Autodesk Fusion 360 part; units mm, degrees
(part 2 of 2)
sketch "Sketch6" plane through (0, 0, 0) normal (0, 0, -1) x (1, 0, 0)
  line L0 (39, 37.5) -> (39, -37.5)
  line L1 (29, -37.5) -> (29, 37.5)
  circle A0 centre (109.2154, 0) radius 7
  circle A1 centre (-109.2154, 0) radius 7
  circle A2 centre (54.6077, 94.5833) radius 7
  circle A3 centre (54.6077, -94.5833) radius 7
  circle A4 centre (-54.6077, -94.5833) radius 7
  circle A5 centre (-54.6077, 94.5833) radius 7
  line L2 (54.6077, 109.3333) -> (-54.6077, 109.3333)
  arc A6 (-54.6077, 109.3333) -> (-67.3816, 101.9583) centre (-54.6077, 94.5833) ccw
  line L3 (-67.3816, 101.9583) -> (-121.9893, 7.375)
  arc A7 (-121.9893, 7.375) -> (-121.9893, -7.375) centre (-109.2154, 0) ccw
  line L4 (-121.9893, -7.375) -> (-67.3816, -101.9583)
  arc A8 (-67.3816, -101.9583) -> (-54.6077, -109.3333) centre (-54.6077, -94.5833) ccw
  line L5 (-54.6077, -109.3333) -> (54.6077, -109.3333)
  arc A9 (54.6077, -109.3333) -> (67.3816, -101.9583) centre (54.6077, -94.5833) ccw
  line L6 (67.3816, -101.9583) -> (121.9893, -7.375)
  arc A10 (121.9893, -7.375) -> (121.9893, 7.375) centre (109.2154, 0) ccw
  line L7 (121.9893, 7.375) -> (67.3816, 101.9583)
  arc A11 (67.3816, 101.9583) -> (54.6077, 109.3333) centre (54.6077, 94.5833) ccw
  line L8 (0, 0) -> (-123.9654, 0) construction
  circle A12 centre (-89.2154, 0) radius 2.35
  line L9 (-53.7561, -78.4378) -> (-50.1995, -84.598)
  arc A13 (-48.1643, -68.6025) -> (-50.3294, -69.8525) centre (-48.1643, -71.1025) ccw
  line L10 (-39.0159, -84.598) -> (-35.4593, -78.4378)
  arc A14 (-41.0511, -85.923) -> (-38.886, -84.673) centre (-41.0511, -83.423) ccw
  line L11 (-48.1643, -85.923) -> (-41.0511, -85.923)
  arc A15 (-53.7561, -76.0878) -> (-53.7561, -78.4378) centre (-51.7209, -77.2628) ccw
  arc A16 (-41.0511, -85.773) -> (-39.0159, -84.598) centre (-41.0511, -83.423) ccw
  line L12 (-41.0511, -68.7525) -> (-48.1643, -68.7525)
  line L13 (-53.886, -78.5128) -> (-50.3294, -84.673)
  line L14 (-35.3294, -76.0128) -> (-38.886, -69.8525)
  arc A17 (-35.3294, -78.5128) -> (-35.3294, -76.0128) centre (-37.4944, -77.2628) ccw
  arc A18 (-38.886, -69.8525) -> (-41.0511, -68.6025) centre (-41.0511, -71.1025) ccw
  circle A19 centre (-32.4026, -66.1229) radius 2.85
  line L15 (-35.4593, -76.0878) -> (-39.0159, -69.9275)
  line L16 (-48.1643, -85.773) -> (-41.0511, -85.773)
  circle A20 centre (-44.6077, -77.2628) radius 2.35
  arc A21 (-35.4593, -78.4378) -> (-35.4593, -76.0878) centre (-37.4944, -77.2628) ccw
  arc A22 (-50.3294, -84.673) -> (-48.1643, -85.923) centre (-48.1643, -83.423) ccw
  arc A23 (-53.886, -76.0128) -> (-53.886, -78.5128) centre (-51.7209, -77.2628) ccw
  line L17 (-38.886, -84.673) -> (-35.3294, -78.5128)
  line L18 (-50.1995, -69.9275) -> (-53.7561, -76.0878)
  arc A24 (-39.0159, -69.9275) -> (-41.0511, -68.7525) centre (-41.0511, -71.1025) ccw
  arc A25 (-48.1643, -68.7525) -> (-50.1995, -69.9275) centre (-48.1643, -71.1025) ccw
  line L19 (-50.3294, -69.8525) -> (-53.886, -76.0128)
  line L20 (-41.0511, -68.6025) -> (-48.1643, -68.6025)
  arc A26 (-50.1995, -84.598) -> (-48.1643, -85.773) centre (-48.1643, -83.423) ccw
  circle A27 centre (-41.0628, -61.1229) radius 2.85
  line L21 (41.0511, -85.773) -> (48.1643, -85.773)
  arc A28 (35.3294, -76.0128) -> (35.3294, -78.5128) centre (37.4944, -77.2628) ccw
  line L22 (53.7561, -76.0878) -> (50.1995, -69.9275)
  arc A29 (53.886, -78.5128) -> (53.886, -76.0128) centre (51.7209, -77.2628) ccw
  line L23 (50.3294, -84.673) -> (53.886, -78.5128)
  arc A30 (39.0159, -84.598) -> (41.0511, -85.773) centre (41.0511, -83.423) ccw
  arc A31 (53.7561, -78.4378) -> (53.7561, -76.0878) centre (51.7209, -77.2628) ccw
  line L24 (39.0159, -69.9275) -> (35.4593, -76.0878)
  line L25 (41.0511, -85.923) -> (48.1643, -85.923)
  line L26 (48.1643, -68.6025) -> (41.0511, -68.6025)
  arc A32 (50.3294, -69.8525) -> (48.1643, -68.6025) centre (48.1643, -71.1025) ccw
  arc A33 (41.0511, -68.6025) -> (38.886, -69.8525) centre (41.0511, -71.1025) ccw
  circle A34 centre (41.0628, -61.1229) radius 2.85
  line L27 (48.1643, -68.7525) -> (41.0511, -68.7525)
  line L28 (50.1995, -84.598) -> (53.7561, -78.4378)
  circle A35 centre (44.6077, -77.2628) radius 2.35
  arc A36 (50.1995, -69.9275) -> (48.1643, -68.7525) centre (48.1643, -71.1025) ccw
  arc A37 (48.1643, -85.923) -> (50.3294, -84.673) centre (48.1643, -83.423) ccw
  arc A38 (38.886, -84.673) -> (41.0511, -85.923) centre (41.0511, -83.423) ccw
  line L29 (53.886, -76.0128) -> (50.3294, -69.8525)
  line L30 (35.4593, -78.4378) -> (39.0159, -84.598)
  arc A39 (41.0511, -68.7525) -> (39.0159, -69.9275) centre (41.0511, -71.1025) ccw
  arc A40 (35.4593, -76.0878) -> (35.4593, -78.4378) centre (37.4944, -77.2628) ccw
  line L31 (35.3294, -78.5128) -> (38.886, -84.673)
  line L32 (38.886, -69.8525) -> (35.3294, -76.0128)
  arc A41 (48.1643, -85.773) -> (50.1995, -84.598) centre (48.1643, -83.423) ccw
  circle A42 centre (32.4026, -66.1229) radius 2.85
  line L33 (94.8072, -7.3353) -> (98.3638, -1.175)
  arc A43 (83.4937, -7.4103) -> (85.6588, -8.6603) centre (85.6588, -6.1603) ccw
  line L34 (92.772, 8.5103) -> (85.6588, 8.5103)
  arc A44 (94.9371, 7.4103) -> (92.772, 8.6603) centre (92.772, 6.1603) ccw
  line L35 (98.4937, 1.25) -> (94.9371, 7.4103)
  arc A45 (92.772, -8.5103) -> (94.8072, -7.3353) centre (92.772, -6.1603) ccw
  arc A46 (94.8072, 7.3353) -> (92.772, 8.5103) centre (92.772, 6.1603) ccw
  line L36 (80.067, -1.175) -> (83.6236, -7.3353)
  line L37 (94.9371, -7.4103) -> (98.4937, -1.25)
  line L38 (83.4937, 7.4103) -> (79.9371, 1.25)
  arc A47 (85.6588, 8.6603) -> (83.4937, 7.4103) centre (85.6588, 6.1603) ccw
  arc A48 (79.9371, 1.25) -> (79.9371, -1.25) centre (82.1021, 0) ccw
  circle A49 centre (73.4654, 5) radius 2.85
  line L39 (83.6236, 7.3353) -> (80.067, 1.175)
  line L40 (98.3638, 1.175) -> (94.8072, 7.3353)
  circle A50 centre (89.2154, 0) radius 2.35
  arc A51 (85.6588, 8.5103) -> (83.6236, 7.3353) centre (85.6588, 6.1603) ccw
  arc A52 (98.4937, -1.25) -> (98.4937, 1.25) centre (96.3286, 0) ccw
  arc A53 (92.772, -8.6603) -> (94.9371, -7.4103) centre (92.772, -6.1603) ccw
  line L41 (92.772, 8.6603) -> (85.6588, 8.6603)
  line L42 (85.6588, -8.5103) -> (92.772, -8.5103)
  arc A54 (80.067, 1.175) -> (80.067, -1.175) centre (82.1021, 0) ccw
  arc A55 (83.6236, -7.3353) -> (85.6588, -8.5103) centre (85.6588, -6.1603) ccw
  line L43 (85.6588, -8.6603) -> (92.772, -8.6603)
  line L44 (79.9371, -1.25) -> (83.4937, -7.4103)
  arc A56 (98.3638, -1.175) -> (98.3638, 1.175) centre (96.3286, 0) ccw
  circle A57 centre (73.4654, -5) radius 2.85
  line L45 (53.7561, 78.4378) -> (50.1995, 84.598)
  arc A58 (48.1643, 68.6025) -> (50.3294, 69.8525) centre (48.1643, 71.1025) ccw
  line L46 (39.0159, 84.598) -> (35.4593, 78.4378)
  arc A59 (41.0511, 85.923) -> (38.886, 84.673) centre (41.0511, 83.423) ccw
  line L47 (48.1643, 85.923) -> (41.0511, 85.923)
  arc A60 (53.7561, 76.0878) -> (53.7561, 78.4378) centre (51.7209, 77.2628) ccw
  arc A61 (41.0511, 85.773) -> (39.0159, 84.598) centre (41.0511, 83.423) ccw
  line L48 (41.0511, 68.7525) -> (48.1643, 68.7525)
  line L49 (53.886, 78.5128) -> (50.3294, 84.673)
  line L50 (35.3294, 76.0128) -> (38.886, 69.8525)
  arc A62 (35.3294, 78.5128) -> (35.3294, 76.0128) centre (37.4944, 77.2628) ccw
  arc A63 (38.886, 69.8525) -> (41.0511, 68.6025) centre (41.0511, 71.1025) ccw
  circle A64 centre (32.4026, 66.1229) radius 2.85
  line L51 (35.4593, 76.0878) -> (39.0159, 69.9275)
  line L52 (48.1643, 85.773) -> (41.0511, 85.773)
  circle A65 centre (44.6077, 77.2628) radius 2.35
  arc A66 (35.4593, 78.4378) -> (35.4593, 76.0878) centre (37.4944, 77.2628) ccw
  arc A67 (50.3294, 84.673) -> (48.1643, 85.923) centre (48.1643, 83.423) ccw
  arc A68 (53.886, 76.0128) -> (53.886, 78.5128) centre (51.7209, 77.2628) ccw
  line L53 (38.886, 84.673) -> (35.3294, 78.5128)
  line L54 (50.1995, 69.9275) -> (53.7561, 76.0878)
  arc A69 (39.0159, 69.9275) -> (41.0511, 68.7525) centre (41.0511, 71.1025) ccw
  arc A70 (48.1643, 68.7525) -> (50.1995, 69.9275) centre (48.1643, 71.1025) ccw
  line L55 (50.3294, 69.8525) -> (53.886, 76.0128)
  line L56 (41.0511, 68.6025) -> (48.1643, 68.6025)
  arc A71 (50.1995, 84.598) -> (48.1643, 85.773) centre (48.1643, 83.423) ccw
  circle A72 centre (41.0628, 61.1229) radius 2.85
  line L57 (-41.0511, 85.773) -> (-48.1643, 85.773)
  arc A73 (-35.3294, 76.0128) -> (-35.3294, 78.5128) centre (-37.4944, 77.2628) ccw
  line L58 (-53.7561, 76.0878) -> (-50.1995, 69.9275)
  arc A74 (-53.886, 78.5128) -> (-53.886, 76.0128) centre (-51.7209, 77.2628) ccw
  line L59 (-50.3294, 84.673) -> (-53.886, 78.5128)
  arc A75 (-39.0159, 84.598) -> (-41.0511, 85.773) centre (-41.0511, 83.423) ccw
  arc A76 (-53.7561, 78.4378) -> (-53.7561, 76.0878) centre (-51.7209, 77.2628) ccw
  line L60 (-39.0159, 69.9275) -> (-35.4593, 76.0878)
  line L61 (-41.0511, 85.923) -> (-48.1643, 85.923)
  line L62 (-48.1643, 68.6025) -> (-41.0511, 68.6025)
  arc A77 (-50.3294, 69.8525) -> (-48.1643, 68.6025) centre (-48.1643, 71.1025) ccw
  arc A78 (-41.0511, 68.6025) -> (-38.886, 69.8525) centre (-41.0511, 71.1025) ccw
  circle A79 centre (-41.0628, 61.1229) radius 2.85
  line L63 (-48.1643, 68.7525) -> (-41.0511, 68.7525)
  line L64 (-50.1995, 84.598) -> (-53.7561, 78.4378)
  circle A80 centre (-44.6077, 77.2628) radius 2.35
  arc A81 (-50.1995, 69.9275) -> (-48.1643, 68.7525) centre (-48.1643, 71.1025) ccw
  arc A82 (-48.1643, 85.923) -> (-50.3294, 84.673) centre (-48.1643, 83.423) ccw
  arc A83 (-38.886, 84.673) -> (-41.0511, 85.923) centre (-41.0511, 83.423) ccw
  line L65 (-53.886, 76.0128) -> (-50.3294, 69.8525)
  line L66 (-35.4593, 78.4378) -> (-39.0159, 84.598)
  arc A84 (-41.0511, 68.7525) -> (-39.0159, 69.9275) centre (-41.0511, 71.1025) ccw
  arc A85 (-35.4593, 76.0878) -> (-35.4593, 78.4378) centre (-37.4944, 77.2628) ccw
  line L67 (-35.3294, 78.5128) -> (-38.886, 84.673)
  line L68 (-38.886, 69.8525) -> (-35.3294, 76.0128)
  arc A86 (-48.1643, 85.773) -> (-50.1995, 84.598) centre (-48.1643, 83.423) ccw
  circle A87 centre (-32.4026, 66.1229) radius 2.85
  circle A88 centre (-89.2154, 0) radius 1.75
  circle A89 centre (0, 0) radius 1.5
  line L69 (-93.947, 8.1954) -> (-84.4838, -8.1954) construction
  line L70 (-84.4838, 8.1954) -> (-93.947, -8.1954) construction
  line L71 (-98.0607, -1) -> (-94.5041, -7.1603)
  arc A90 (-94.5041, -7.1603) -> (-92.772, -8.1603) centre (-92.772, -6.1603) ccw
  line L72 (-92.772, -8.1603) -> (-85.6588, -8.1603)
  arc A91 (-85.6588, -8.1603) -> (-83.9267, -7.1603) centre (-85.6588, -6.1603) ccw
  line L73 (-83.9267, -7.1603) -> (-80.3701, -1)
  arc A92 (-80.3701, -1) -> (-80.3701, 1) centre (-82.1021, 0) ccw
  line L74 (-80.3701, 1) -> (-83.9267, 7.1603)
  arc A93 (-83.9267, 7.1603) -> (-85.6588, 8.1603) centre (-85.6588, 6.1603) ccw
  line L75 (-85.6588, 8.1603) -> (-92.772, 8.1603)
  arc A94 (-92.772, 8.1603) -> (-94.5041, 7.1603) centre (-92.772, 6.1603) ccw
  line L76 (-94.5041, 7.1603) -> (-98.0607, 1)
  arc A95 (-98.0607, 1) -> (-98.0607, -1) centre (-96.3286, 0) ccw
  arc A96 (39, 37.5) -> (29, 37.5) centre (34, 37.5) ccw
  arc A97 (29, -37.5) -> (39, -37.5) centre (34, -37.5) ccw
  circle A98 centre (73.4654, 5) radius 2.85
  circle A99 centre (-32.4026, -66.1229) radius 2.85
  circle A100 centre (-73.4654, -5) radius 2.85
  circle A101 centre (-41.0628, 61.1229) radius 2.85
  circle A102 centre (32.4026, -66.1229) radius 2.85
  circle A103 centre (41.0628, 61.1229) radius 2.85
  circle A104 centre (73.4654, -5) radius 2.85
  circle A105 centre (-41.0628, -61.1229) radius 2.85
  circle A106 centre (-73.4654, 5) radius 2.85
  circle A107 centre (-32.4026, 66.1229) radius 2.85
  circle A108 centre (41.0628, -61.1229) radius 2.85
  circle A109 centre (32.4026, 66.1229) radius 2.85
  line L77 (-94.9371, 7.4103) -> (-98.4937, 1.25)
  arc A110 (-98.4937, 1.25) -> (-98.4937, -1.25) centre (-96.3286, 0) ccw
  line L78 (-98.4937, -1.25) -> (-94.9371, -7.4103)
  arc A111 (-94.9371, -7.4103) -> (-92.772, -8.6603) centre (-92.772, -6.1603) ccw
  line L79 (-92.772, -8.6603) -> (-85.6588, -8.6603)
  arc A112 (-85.6588, -8.6603) -> (-83.4937, -7.4103) centre (-85.6588, -6.1603) ccw
  line L80 (-83.4937, -7.4103) -> (-79.9371, -1.25)
  arc A113 (-79.9371, -1.25) -> (-79.9371, 1.25) centre (-82.1021, 0) ccw
  line L81 (-79.9371, 1.25) -> (-83.4937, 7.4103)
  arc A114 (-83.4937, 7.4103) -> (-85.6588, 8.6603) centre (-85.6588, 6.1603) ccw
  line L82 (-85.6588, 8.6603) -> (-92.772, 8.6603)
  arc A115 (-92.772, 8.6603) -> (-94.9371, 7.4103) centre (-92.772, 6.1603) ccw
  arc A116 (-50.3294, -84.673) -> (-48.1643, -85.923) centre (-48.1643, -83.423) ccw
  line L83 (-48.1643, -85.923) -> (-41.0511, -85.923)
  arc A117 (-41.0511, -85.923) -> (-38.886, -84.673) centre (-41.0511, -83.423) ccw
  line L84 (-38.886, -84.673) -> (-35.3294, -78.5128)
  arc A118 (-35.3294, -78.5128) -> (-35.3294, -76.0128) centre (-37.4944, -77.2628) ccw
  line L85 (-35.3294, -76.0128) -> (-38.886, -69.8525)
  arc A119 (-38.886, -69.8525) -> (-41.0511, -68.6025) centre (-41.0511, -71.1025) ccw
  line L86 (-41.0511, -68.6025) -> (-48.1643, -68.6025)
  arc A120 (-48.1643, -68.6025) -> (-50.3294, -69.8525) centre (-48.1643, -71.1025) ccw
  line L87 (-53.886, -78.5128) -> (-50.3294, -84.673)
  arc A121 (-53.886, -76.0128) -> (-53.886, -78.5128) centre (-51.7209, -77.2628) ccw
  line L88 (-50.3294, -69.8525) -> (-53.886, -76.0128)
  arc A122 (48.1643, -85.923) -> (50.3294, -84.673) centre (48.1643, -83.423) ccw
  line L89 (50.3294, -84.673) -> (53.886, -78.5128)
  arc A123 (53.886, -78.5128) -> (53.886, -76.0128) centre (51.7209, -77.2628) ccw
  line L90 (53.886, -76.0128) -> (50.3294, -69.8525)
  arc A124 (50.3294, -69.8525) -> (48.1643, -68.6025) centre (48.1643, -71.1025) ccw
  line L91 (48.1643, -68.6025) -> (41.0511, -68.6025)
  arc A125 (41.0511, -68.6025) -> (38.886, -69.8525) centre (41.0511, -71.1025) ccw
  line L92 (38.886, -69.8525) -> (35.3294, -76.0128)
  arc A126 (35.3294, -76.0128) -> (35.3294, -78.5128) centre (37.4944, -77.2628) ccw
  line L93 (41.0511, -85.923) -> (48.1643, -85.923)
  arc A127 (38.886, -84.673) -> (41.0511, -85.923) centre (41.0511, -83.423) ccw
  line L94 (35.3294, -78.5128) -> (38.886, -84.673)
  arc A128 (98.4937, -1.25) -> (98.4937, 1.25) centre (96.3286, 0) ccw
  line L95 (98.4937, 1.25) -> (94.9371, 7.4103)
  arc A129 (94.9371, 7.4103) -> (92.772, 8.6603) centre (92.772, 6.1603) ccw
  line L96 (92.772, 8.6603) -> (85.6588, 8.6603)
  arc A130 (85.6588, 8.6603) -> (83.4937, 7.4103) centre (85.6588, 6.1603) ccw
  line L97 (83.4937, 7.4103) -> (79.9371, 1.25)
  arc A131 (79.9371, 1.25) -> (79.9371, -1.25) centre (82.1021, 0) ccw
  line L98 (79.9371, -1.25) -> (83.4937, -7.4103)
  arc A132 (83.4937, -7.4103) -> (85.6588, -8.6603) centre (85.6588, -6.1603) ccw
  line L99 (94.9371, -7.4103) -> (98.4937, -1.25)
  arc A133 (92.772, -8.6603) -> (94.9371, -7.4103) centre (92.772, -6.1603) ccw
  line L100 (85.6588, -8.6603) -> (92.772, -8.6603)
  arc A134 (50.3294, 84.673) -> (48.1643, 85.923) centre (48.1643, 83.423) ccw
  line L101 (48.1643, 85.923) -> (41.0511, 85.923)
  arc A135 (41.0511, 85.923) -> (38.886, 84.673) centre (41.0511, 83.423) ccw
  line L102 (38.886, 84.673) -> (35.3294, 78.5128)
  arc A136 (35.3294, 78.5128) -> (35.3294, 76.0128) centre (37.4944, 77.2628) ccw
  line L103 (35.3294, 76.0128) -> (38.886, 69.8525)
  arc A137 (38.886, 69.8525) -> (41.0511, 68.6025) centre (41.0511, 71.1025) ccw
  line L104 (41.0511, 68.6025) -> (48.1643, 68.6025)
  arc A138 (48.1643, 68.6025) -> (50.3294, 69.8525) centre (48.1643, 71.1025) ccw
  line L105 (53.886, 78.5128) -> (50.3294, 84.673)
  arc A139 (53.886, 76.0128) -> (53.886, 78.5128) centre (51.7209, 77.2628) ccw
  line L106 (50.3294, 69.8525) -> (53.886, 76.0128)
  arc A140 (-48.1643, 85.923) -> (-50.3294, 84.673) centre (-48.1643, 83.423) ccw
  line L107 (-50.3294, 84.673) -> (-53.886, 78.5128)
  arc A141 (-53.886, 78.5128) -> (-53.886, 76.0128) centre (-51.7209, 77.2628) ccw
  line L108 (-53.886, 76.0128) -> (-50.3294, 69.8525)
  arc A142 (-50.3294, 69.8525) -> (-48.1643, 68.6025) centre (-48.1643, 71.1025) ccw
  line L109 (-48.1643, 68.6025) -> (-41.0511, 68.6025)
  arc A143 (-41.0511, 68.6025) -> (-38.886, 69.8525) centre (-41.0511, 71.1025) ccw
  line L110 (-38.886, 69.8525) -> (-35.3294, 76.0128)
  arc A144 (-35.3294, 76.0128) -> (-35.3294, 78.5128) centre (-37.4944, 77.2628) ccw
  line L111 (-41.0511, 85.923) -> (-48.1643, 85.923)
  arc A145 (-38.886, 84.673) -> (-41.0511, 85.923) centre (-41.0511, 83.423) ccw
  line L112 (-35.3294, 78.5128) -> (-38.886, 84.673)
  circle A146 centre (-0.25, 75.9996) radius 2.85
  point P0 (-79.2154, 0)
  point P1 (-98.9654, 0)
  point P2 (-89.2154, 0)
  point P3 (-39.6077, -68.6025)
  point P4 (-49.6077, -85.923)
  point P5 (-44.6077, -77.2628)
  point P6 (39.6077, -68.6025)
  point P7 (49.6077, -85.923)
  point P8 (44.6077, -77.2628)
  point P9 (79.2154, 0)
  point P10 (99.2154, 0)
  point P11 (89.2154, 0)
  point P12 (39.6077, 68.6025)
  point P13 (49.6077, 85.923)
  point P14 (44.6077, 77.2628)
  point P15 (-39.6077, 68.6025)
  point P16 (-49.6077, 85.923)
  point P17 (-44.6077, 77.2628)
  dimension "d112" = 25
  dimension "d115" = 4.7
  dimension "d118" = 3.5
  dimension "d124" = 3
  dimension "d159" = 0.5
  dimension "d161" = 360
  constraint coincident L8.start A89.centre
  constraint midpoint A7 L8.end
  constraint coincident L8 P2
  constraint coincident P2 A12.centre
  constraint concentric A12 A88
  constraint tangent L76 A95
  constraint tangent L73 A92
  constraint tangent A94 L76
  constraint tangent L71 A90
  constraint tangent L75 A94
  constraint tangent L71 A95
  constraint tangent A90 L72
  constraint tangent L74 A93
  constraint tangent A93 L75
  constraint tangent A91 L73
  constraint tangent L72 A91
  constraint tangent A92 L74
  measures "d112" distance of L8.end P1
  measures "d115" diameter of A12
  measures "d118" diameter of A88
  measures "d124" diameter of A89
extrude "Extrude16" add sketch "Sketch6" along normal blind 5 separate body contours A12 | L71 A90 L72 A91 L73 A92 L74 A93 L75 A94 L76 A95 makes body 3
extrude "Extrude17" cut sketch "Sketch6" against normal blind 4.2 contours A12 | A20 | A35 | A50 | A65 | A80 | A88 bodies 1
chamfer "Chamfer3" distance 1.5 angle 45 1 edges at (-90.847, -0.6328, -5) on bodies 3
sketch "Sketch7" plane through (0, 0, 0) normal (0, 0, -1) x (1, 0, 0)
  circle A0 centre (44.6077, 77.2628) radius 2.35
  circle A1 centre (-44.6077, -77.2628) radius 2.35
  circle A2 centre (89.2154, 0) radius 2.35
  circle A3 centre (-44.6077, 77.2628) radius 2.35
  circle A4 centre (-89.2154, 0) radius 2.35
  circle A5 centre (44.6077, -77.2628) radius 2.35
  line L0 (39, 37.5) -> (39, -37.5)
  line L1 (29, -37.5) -> (29, 37.5)
  circle A6 centre (109.2154, 0) radius 7
  circle A7 centre (-109.2154, 0) radius 7
  circle A8 centre (54.6077, 94.5833) radius 7
  circle A9 centre (54.6077, -94.5833) radius 7
  circle A10 centre (-54.6077, -94.5833) radius 7
  circle A11 centre (-54.6077, 94.5833) radius 7
  line L2 (54.6077, 109.3333) -> (-54.6077, 109.3333)
  arc A12 (-54.6077, 109.3333) -> (-67.3816, 101.9583) centre (-54.6077, 94.5833) ccw
  line L3 (-67.3816, 101.9583) -> (-121.9893, 7.375)
  arc A13 (-121.9893, 7.375) -> (-121.9893, -7.375) centre (-109.2154, 0) ccw
  line L4 (-121.9893, -7.375) -> (-67.3816, -101.9583)
  arc A14 (-67.3816, -101.9583) -> (-54.6077, -109.3333) centre (-54.6077, -94.5833) ccw
  line L5 (-54.6077, -109.3333) -> (54.6077, -109.3333)
  arc A15 (54.6077, -109.3333) -> (67.3816, -101.9583) centre (54.6077, -94.5833) ccw
  line L6 (67.3816, -101.9583) -> (121.9893, -7.375)
  arc A16 (121.9893, -7.375) -> (121.9893, 7.375) centre (109.2154, 0) ccw
  line L7 (121.9893, 7.375) -> (67.3816, 101.9583)
  arc A17 (67.3816, 101.9583) -> (54.6077, 109.3333) centre (54.6077, 94.5833) ccw
  circle A18 centre (-71.8801, 41.5) radius 2.25
  circle A19 centre (71.8801, 41.5) radius 2.25
  circle A20 centre (0, -83) radius 2.25
  circle A21 centre (-71.8801, 41.5) radius 2.25
  arc A22 (39, 37.5) -> (29, 37.5) centre (34, 37.5) ccw
  arc A23 (29, -37.5) -> (39, -37.5) centre (34, -37.5) ccw
  circle A24 centre (73.4654, 5) radius 2.85
  circle A25 centre (-32.4026, -66.1229) radius 2.85
  circle A26 centre (-73.4654, -5) radius 2.85
  circle A27 centre (-41.0628, 61.1229) radius 2.85
  circle A28 centre (32.4026, -66.1229) radius 2.85
  circle A29 centre (41.0628, 61.1229) radius 2.85
  circle A30 centre (73.4654, -5) radius 2.85
  circle A31 centre (-41.0628, -61.1229) radius 2.85
  circle A32 centre (-73.4654, 5) radius 2.85
  circle A33 centre (-32.4026, 66.1229) radius 2.85
  circle A34 centre (41.0628, -61.1229) radius 2.85
  circle A35 centre (32.4026, 66.1229) radius 2.85
  circle A36 centre (-0.25, 75.9996) radius 2.85
  dimension "d127" = 4.5
  dimension "d128" = 4.5
  dimension "d129" = 4.5
  dimension "d156" = 83
  dimension "d157" = 83
  dimension "d158" = 83
  constraint concentric A18 A21
  measures "d127" diameter of A18
  measures "d128" diameter of A19
  measures "d129" diameter of A20
  measures "d156" distance of A20.centre origin
  measures "d157" distance of A18.centre origin
  measures "d158" distance of A19.centre origin
extrude "Extrude19" cut sketch "Sketch7" against normal blind 4 contours A18 A21 | A19 | A20 bodies 1
copy_body "Body->Comp1" bodies 3 removing the originals makes body 4 in component "foot"
component "foot" placed x (1, 0, 0) y (0, 1, 0) z (0, 0, 1) at (0, 0, 0)
hidden bodies 4
equation "d1 = base_diameter / 2"
equation "base_diameter = 260 mm"
equation "d3 = base_height"
equation "base_height = 6.5 mm"
equation "d19 = -base_height"
equation "d21 = -base_height"
equation "d25 = base_height / 2"
equation "d37 = -base_height"
equation "internal_height = 90 mm"
equation "d54 = internal_height"
equation "d56 = internal_height"
equation "d82 = -base_height"
equation "d92 = 3.15 mm + ( 5.7 / 2 ) * 1 mm"
equation "d93 = 68.15 mm + ( 5.7 / 2 ) * 1 mm"
equation "d149 = -base_height"
equation "d152 = -base_height"
named bodies: "Base", "foot", "Battery Stop"

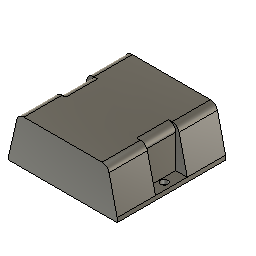
design "buck_converter_30a"
Autodesk Fusion 360 part; units mm, degrees
sketch "Sketch1" plane through (0, 0, 0) normal (0, 0, 1) x (1, 0, 0)
  line L0 (37.5, -37.5) -> (-37.5, -37.5)
  line L1 (-37.5, -37.5) -> (-37.5, 37.5)
  line L2 (-37.5, 37.5) -> (37.5, 37.5)
  line L3 (37.5, 37.5) -> (37.5, -37.5)
  line L4 (37.5, -37.5) -> (-37.5, 37.5) construction
  line L5 (-37.5, -37.5) -> (37.5, 37.5) construction
  line L6 (0, 0) -> (32.5, 0)
  circle A0 centre (32.5, 0) radius 2.5
  line L7 (0, 0) -> (0, -9.2725)
  circle A1 centre (-32.5, 0) radius 2.5
  line L8 (29.5, -11) -> (37.5, -11)
  line L9 (37.5, -11) -> (37.5, 11)
  line L10 (37.5, 11) -> (29.5, 11)
  line L11 (29.5, 11) -> (29.5, -11)
  line L12 (33.5, 11) -> (33.5, 37.5) construction
  line L13 (33.5, -11) -> (33.5, -37.5) construction
  line L14 (-37.5, -11) -> (-37.5, 11)
  line L15 (-37.5, 11) -> (-29.5, 11)
  line L16 (-29.5, -11) -> (-37.5, -11)
  line L17 (-29.5, 11) -> (-29.5, -11)
  dimension "d1" = 75
  dimension "d2" = 75
  dimension "d3" = 32.5
  dimension "d4" = 5
  dimension "d5" = 8
  dimension "d6" = 22
  constraint horizontal L0
  constraint perpendicular L0 L1
  constraint parallel L0 L2
  constraint parallel L1 L3
  constraint coincident L4 L6.start
  constraint coincident L5 L6.start
  constraint coincident L6.start L7.start
  constraint horizontal L6
  constraint coincident L6.end A0.centre
  constraint perpendicular L6 L7
  constraint symmetric A0 L7 A1
  constraint horizontal L8
  constraint vertical L9
  constraint horizontal L10
  constraint vertical L11
  constraint midpoint L10 L12.start
  constraint coincident L2 L12.end
  constraint perpendicular L2 L12
  constraint midpoint L8 L13.start
  constraint coincident L0 L13.end
  constraint perpendicular L0 L13
  constraint equal L12 L13
  constraint coincident L3 L8.end
  constraint symmetric L7 L8.start L16.start
  constraint symmetric L7 L8.end L14.start
  constraint symmetric L7 L9.end L14.end
  constraint symmetric L7 L10.end L15.end
  measures "d1" distance of L1.end L2.end
  measures "d2" distance of L0.end L1.end
  measures "d3" distance of L6.start L6.end
  measures "d4" diameter of A0
  measures "d5" distance of L8.start L8.end
  measures "d6" distance of L8.start L10.end
extrude "Extrude1" add sketch "Sketch1" along normal blind 31 contours L0 L1 L2 L3 L8 L10 L11 L15 L16 L17
extrude "Extrude2" add sketch "Sketch1" along normal blind 3 contours L3 L8 L9 L10 L11 | L1 L14 L15 L16 L17
chamfer "Chamfer1" distance 6.5 distance2 28 4 edges at (-37.5, 24.25, 31) (-37.5, -24.25, 31) (37.5, -24.25, 31) (37.5, 24.25, 31) measured on face at (-9.8333, 28.6667, 31) measured on face at (-9.8333, 28.6667, 31) measured on face at (-9.8333, 28.6667, 31) measured on face at (-9.8333, 28.6667, 31)
sketch "Sketch2" plane through (0, 37.5, 0) normal (0, 1, 0) x (-1, 0, 0)
  line L0 (-31, 31) -> (-37.5, 3)
  line L1 (-37.5, 3) -> (-37.5, 0)
  line L2 (-37.5, 0) -> (37.5, 0)
  line L3 (37.5, 0) -> (37.5, 3)
  line L4 (37.5, 3) -> (31, 31)
  line L5 (31, 31) -> (-31, 31)
  line L6 (-15, 10) -> (15, 10)
  line L7 (15, 10) -> (15, -10)
  line L8 (15, -10) -> (-15, -10)
  line L9 (-15, -10) -> (-15, 10)
  line L10 (-15, 10) -> (15, -10) construction
  line L11 (15, 10) -> (-15, -10) construction
  dimension "d13" = 30
  dimension "d14" = 20
  constraint horizontal L6
  constraint perpendicular L6 L7
  constraint parallel L6 L8
  constraint parallel L7 L9
  constraint coincident L10 origin
  constraint coincident L11 origin
  measures "d13" distance of L7.end L8.end
  measures "d14" distance of L6.end L7.end
extrude "Extrude3" add sketch "Sketch2" along normal blind 15 contours L2 L6 L7 L9
fillet "Fillet1" radius 5 4 edges at (-15, 45, 10) (-15, 45, 0) (15, 45, 10) (15, 45, 0)
fillet "Fillet2" radius 5 6 edges at (-31, 24.25, 31) (-31, -24.25, 31) (-29.5, 0, 31) (31, -24.25, 31) (29.5, 0, 31) (31, 24.25, 31)
